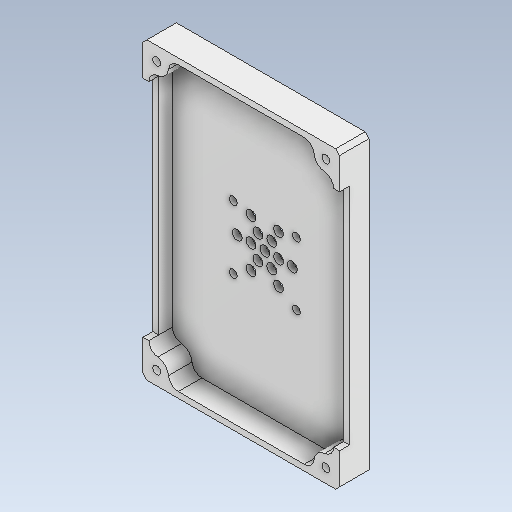
# Autodesk Inventor part: 10-06-019 Capcac Arduino
Saved by Autodesk Inventor 2020 (Build 240168000, 168)
## iProperties
Created: 2020-03-06
Part Number: 10-06-019 Capcac Arduino
Material: ABS Plastic
Document SubType Name: Modeling
Designer: 40743
Density: 1.06 g/cm^3
Appearance: Smooth - White
Mass: 66.0159 g
Surface Area: 413.843 cm^2
Volume: 62.2792 cm^3
Description: Capac Arduino
Author: 40743
Subject: 029
Autodesk Inventor part; units mm, degrees
ref_plane "YZ Plane" through (0, 0, 0) normal (1, 0, 0) x (0, 1, 0)
ref_plane "XZ Plane" through (0, 0, 0) normal (0, 1, 0) x (-1, 0, 0)
ref_plane "XY Plane" through (0, 0, 0) normal (0, 0, 1) x (1, 0, 0)
sketch "Sketch1" plane through (0, 0, 0) normal (0, 0, 1) x (1, 0, 0)
  line L0 (-50, 75) -> (50, 75)
  line L1 (50, 75) -> (50, -75)
  line L2 (50, -75) -> (-50, -75)
  line L3 (-50, -75) -> (-50, 75)
  point P0 (0, 0)
  point P1 (0, 75)
  point P2 (-50, 0)
  dimension "d0" = 100
  dimension "d1" = 150
  constraints: 8 end point, 2 midpoint, 2 parallel, 1 horizontal, 1 horizontal alignment, 1 perpendicular, 1 vertical alignment
  measures "d0" distance of L0.start L0.end
  measures "d1" distance of L2.end L0.start
extrude "Extrusion1" add sketch "Sketch1" along normal blind 15
sketch "Sketch2" plane through (0, 0, 15) normal (0, 0, 1) x (1, 0, 0)
  line L0 (50, 75) -> (-50, 75) projected
  line L1 (-50, 75) -> (-50, -75) projected
  line L2 (-50, -75) -> (50, -75) projected
  line L3 (50, -75) -> (50, 75) projected
  line L4 (47, 72) -> (-47, 72)
  line L5 (-47, 72) -> (-47, -72)
  line L6 (-47, -72) -> (47, -72)
  line L7 (47, -72) -> (47, 72)
  point P0 (0, 0)
  dimension "d4" = 3
  constraints: 8 end point, 3 other
  measures "d4" distance between parallel lines of L7 L3
extrude "Extrusion2" cut sketch "Sketch2" against normal blind 12 contours L7 L6 L5 L4
sketch "Sketch3" plane through (0, 0, 0) normal (0, 0, -1) x (-1, 0, 0)
  line L0 (-43, -68) -> (43, -68) construction
  line L1 (43, -68) -> (43, 68) construction
  line L2 (43, 68) -> (-43, 68) construction
  line L3 (-43, 68) -> (-43, -68) construction
  line L4 (-50, 75) -> (50, 75) construction
  line L5 (-50, -75) -> (-50, 75) construction
  line L6 (50, -75) -> (-50, -75) construction
  line L7 (-47, 72) -> (-47, -72) projected
  line L8 (47, 72) -> (-47, 72) projected
  line L9 (47, -72) -> (47, 72) projected
  line L10 (-47, -72) -> (47, -72) projected
  point P0 (0, 0)
  point P1 (0, 68)
  point P2 (0, 75)
  point P3 (-43, 0)
  point P4 (-50, 0)
  dimension "d17" = 4
  dimension "d18" = 4
  constraints: 8 end point, 4 coincident, 4 midpoint, 2 parallel, 1 horizontal, 1 horizontal alignment, 1 perpendicular, 1 vertical alignment
  measures "d17" distance between parallel lines of L0 L10
  measures "d18" distance between parallel lines of L1 L9
hole "Hole1" at (43, -68, 0) at (43, 68, 0) at (-43, 68, 0) at (-43, -68, 0) direction (0, 0, 1) diameter 4 end through all
sketch "Sketch4" plane through (0, 0, 3) normal (0, 0, 1) x (1, 0, 0)
  circle A0 centre (43, -68) radius 6
  circle A1 centre (43, 68) radius 6
  circle A2 centre (-43, 68) radius 6
  circle A3 centre (-43, -68) radius 6
  circle A4 centre (43, -68) radius 2 projected
  circle A5 centre (-43, -68) radius 2 projected
  circle A6 centre (-43, 68) radius 2 projected
  circle A7 centre (43, 68) radius 2 projected
  point P0 (0, 0)
  point P1 (44.2679, -72)
  point P2 (47, -69.2679)
  dimension "d16" = 12
  constraints: 4 centre point, 3 concentric, 3 equal radius, 2 other
  measures "d16" diameter of A0
extrude "Extrusion3" add sketch "Sketch4" along normal up to surface (12 mm away)
fillet "Fillet1" radius 5 8 edges at (-47, -63.5279, 9) (-38.5279, -72, 9) (-47, 63.5279, 9) (-38.5279, 72, 9) (47, 63.5279, 9) (38.5279, 72, 9) (38.5279, -72, 9) (47, -63.5279, 9)
sketch "Sketch6" plane through (0, 0, 0) normal (1, 0, 0) x (0, 1, 0)
  line L0 (57.0455, 10) -> (-57.0455, 10)
  line L1 (-57.0455, 10) -> (-57.0455, 15)
  line L2 (-57.0455, 15) -> (57.0455, 15)
  line L3 (57.0455, 15) -> (57.0455, 10)
  line L4 (-57.0455, 3) -> (-57.0455, 15) projected
  line L5 (57.0455, 15) -> (57.0455, 3) projected
  line L6 (-75, 0) -> (75, 0) projected
  line L7 (-72, 15) -> (72, 15) projected
  point P0 (0, 0)
  dimension "d24" = 10
  constraints: 8 end point, 3 collinear, 2 parallel, 1 horizontal, 1 perpendicular
  measures "d24" distance between parallel lines of L0 L6
extrude "Extrusion5" cut sketch "Sketch6" against normal through all both and the other way through all
chamfer "Chamfer1" distance 2 angle 45 4 edges at (50, 75, 7.5) (50, -75, 7.5) (-50, -75, 7.5) (-50, 75, 7.5)
sketch "Sketch7" plane through (0, 0, 3) normal (0, 0, 1) x (1, 0, 0)
  line L0 (47, 57.0455) -> (47, -57.0455) projected
  arc A0 (17.7914, 11.7526) -> (13.7247, 15.8193) centre (16.0655, 14.0934) ccw projected
  arc A1 (13.7247, -19.7635) -> (17.7914, -15.6968) centre (16.0655, -18.0376) ccw projected
  arc A2 (-17.7914, -15.6968) -> (-13.7247, -19.7635) centre (-16.0655, -18.0376) ccw projected
  arc A3 (-13.7247, 15.8193) -> (-17.7914, 11.7526) centre (-16.0655, 14.0934) ccw projected
  point P0 (0, 0)
hole "Hole2" at (-16.0655, -18.0376, 3) at (-16.0655, 14.0934, 3) at (16.0655, 14.0934, 3) at (16.0655, -18.0376, 3) direction (0, 0, -1) diameter 4 end through all
sketch "Sketch8" plane through (0, 0, 3) normal (0, 0, 1) x (1, 0, 0)
  circle A0 centre (0, 0) radius 2.5
  circle A1 centre (7, 0) radius 2.5
  circle A2 centre (14, 0) radius 2.5
  dimension "d37" = 5
  dimension "d38" = 7
  dimension "d39" = 7
  constraints: 3 centre point, 2 equal radius, 2 horizontal alignment, 1 coincident
  measures "d37" diameter of A0
  measures "d38" distance of point (0, 0) A1.centre
  measures "d39" distance of A1.centre A2.centre
extrude "Extrusion6" cut sketch "Sketch8" against normal through all
pattern_circular "Circular Pattern1" count 6 over 360 about axis through (0, 0, 3) along (0, 0, -1) of "Extrusion6"
equation "\"d39\" = d38"
body "Solid1"
